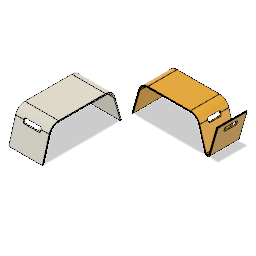
33-Office Desks v1 (Autodesk Fusion 360 design; units mm, degrees)
Autodesk Fusion 360 part; units mm, degrees
sketch "Sketch1" plane through (0, 0, 0) normal (0, 0, 1) x (1, 0, 0)
  line L0 (-100, 0) -> (-84.1445, 55.4944)
  line L1 (-64.914, 70) -> (34.914, 70)
  line L2 (54.1445, 55.4944) -> (68.9639, 3.6264)
  line L3 (73.7715, 0) -> (76.2285, 0)
  line L4 (81.0361, 3.6264) -> (99.8713, 69.5494)
  arc A0 (-64.914, 70) -> (-84.1445, 55.4944) centre (-64.914, 50) ccw
  arc A1 (54.1445, 55.4944) -> (34.914, 70) centre (34.914, 50) ccw
  arc A2 (68.9639, 3.6264) -> (73.7715, 0) centre (73.7715, 5) ccw
  arc A3 (76.2285, 0) -> (81.0361, 3.6264) centre (76.2285, 5) ccw
  line L5 (-102.8846, 0.8242) -> (-87.029, 56.3186)
  arc A4 (-64.914, 73) -> (-87.029, 56.3186) centre (-64.914, 50) ccw
  line L6 (-64.914, 73) -> (34.914, 73)
  arc A5 (57.029, 56.3186) -> (34.914, 73) centre (34.914, 50) ccw
  line L7 (57.029, 56.3186) -> (71.8485, 4.4506)
  arc A6 (71.8485, 4.4506) -> (73.7715, 3) centre (73.7715, 5) ccw
  line L8 (73.7715, 3) -> (76.2285, 3)
  arc A7 (76.2285, 3) -> (78.1515, 4.4506) centre (76.2285, 5) ccw
  line L9 (78.1515, 4.4506) -> (96.9082, 70.0989)
  line L10 (-102.8846, 0.8242) -> (-103.12, 0)
  line L11 (-100, 0) -> (-103.12, 0)
  line L12 (97.8697, 70.8242) -> (98.9097, 70.8242)
  arc A8 (97.8697, 70.8242) -> (96.9082, 70.0989) centre (97.8697, 69.8242) ccw
  arc A9 (99.8713, 69.5494) -> (98.9097, 70.8242) centre (98.9097, 69.8242) ccw
  dimension "d1" = 20
  dimension "d2" = 5
  dimension "d4" = 1
  constraint horizontal L1
  constraint parallel L1 L3
  constraint tangent L0 A0
  constraint tangent L1 A0
  constraint tangent L1 A1
  constraint tangent L2 A1
  constraint equal A0 A1
  constraint tangent L2 A2
  constraint tangent L3 A2
  constraint tangent L3 A3
  constraint tangent L4 A3
  constraint equal A2 A3
  constraint parallel L5 L10
  constraint horizontal L11
  constraint horizontal L12
  constraint parallel L0 L5
  constraint concentric A0 A4
  constraint parallel L1 L6
  constraint concentric A1 A5
  constraint parallel L2 L7
  constraint concentric A2 A6
  constraint parallel L3 L8
  constraint concentric A3 A7
  constraint parallel L4 L9
  constraint tangent A5 L7
  constraint tangent L6 A5
  constraint tangent L5 A4
  constraint tangent A4 L6
  constraint tangent L7 A6
  constraint tangent A6 L8
  constraint tangent L8 A7
  constraint tangent A7 L9
  constraint tangent L9 A8
  constraint tangent L12 A8
  constraint tangent L12 A9
  constraint equal A8 A9
  measures "d1" radius of A0
  measures "d2" radius of A2
  measures "d4" radius of A8
extrude "Extrude1" add sketch "Sketch1" along normal blind 70 makes body 1
sketch "Sketch2" plane through (0, 0, 0) normal (1, 0, 0) x (0, 0, -1)
  line L0 (-22.5, 50) -> (-47.5, 50)
  line L1 (-50, 52.5) -> (-50, 57.5)
  line L2 (-47.5, 60) -> (-22.5, 60)
  line L3 (-20, 57.5) -> (-20, 52.5)
  arc A0 (-47.5, 60) -> (-50, 57.5) centre (-47.5, 57.5) ccw
  arc A1 (-50, 52.5) -> (-47.5, 50) centre (-47.5, 52.5) ccw
  arc A2 (-22.5, 50) -> (-20, 52.5) centre (-22.5, 52.5) ccw
  arc A3 (-20, 57.5) -> (-22.5, 60) centre (-22.5, 57.5) ccw
  dimension "d7" = 2.5
  constraint horizontal L0
  constraint vertical L1
  constraint horizontal L2
  constraint vertical L3
  constraint tangent L1 A0
  constraint tangent L2 A0
  constraint tangent L0 A1
  constraint tangent L1 A1
  constraint equal A0 A1
  constraint tangent L0 A2
  constraint tangent L3 A2
  constraint equal A0 A2
  constraint tangent L2 A3
  constraint tangent L3 A3
  constraint equal A0 A3
  measures "d7" radius of A0
extrude "Extrude2" cut sketch "Sketch2" along normal mid plane 300 bodies 1
fillet "Fillet1" radius 0.5 42 edges at (-95.0745, 28.1593, 0) (-78.7645, 68.362, 0) (-15, 73, 0) (48.7645, 68.362, 0) (64.4387, 30.3846, 0) (72.5671, 3.4033, 0) (75, 3, 0) (77.4329, 3.4033, 0) (87.5299, 37.2747, 0) (97.2675, 70.6225, 0) (98.3897, 70.8242, 0) (99.7081, 70.4264, 0) (90.4537, 36.5879, 0) (79.2395, 1.0083, 0) (75, 0, 0) (70.7605, 1.0083, 0) (61.5542, 29.5604, 0) (46.9579, 65.967, 0) (-15, 70, 0) (-76.9579, 65.967, 0) (-92.0722, 27.7472, 0) (-92.0722, 27.7472, 70) (-76.9579, 65.967, 70) (-15, 70, 70) (46.9579, 65.967, 70) (61.5542, 29.5604, 70) (70.7605, 1.0083, 70) (75, 0, 70) (79.2395, 1.0083, 70) (90.4537, 36.5879, 70) (99.7081, 70.4264, 70) (98.3897, 70.8242, 70) (97.2675, 70.6225, 70) (87.5299, 37.2747, 70) (77.4329, 3.4033, 70) (75, 3, 70) (72.5671, 3.4033, 70) (64.4387, 30.3846, 70) (48.7645, 68.362, 70) (-15, 73, 70) (-78.7645, 68.362, 70) (-95.0745, 28.1593, 70) on bodies 1
sketch "Sketch3" plane through (0, 0, 0) normal (1, 0, 0) x (0, 0, -1)
  line L0 (-220, 0) -> (-204.1445, 55.4944)
  line L1 (-184.914, 70) -> (-74.3884, 70)
  line L2 (-55.158, 55.4944) -> (-39.4041, 0.3558)
  arc A0 (-184.914, 70) -> (-204.1445, 55.4944) centre (-184.914, 50) ccw
  arc A1 (-55.158, 55.4944) -> (-74.3884, 70) centre (-74.3884, 50) ccw
  line L3 (-222.8846, 0.8242) -> (-207.029, 56.3186)
  arc A2 (-184.914, 73) -> (-207.029, 56.3186) centre (-184.914, 50) ccw
  line L4 (-184.914, 73) -> (-74.3884, 73)
  arc A3 (-52.2734, 56.3186) -> (-74.3884, 73) centre (-74.3884, 50) ccw
  line L5 (-52.2734, 56.3186) -> (-36.5195, 1.1799)
  line L6 (-222.8846, 0.8242) -> (-223.12, 0)
  line L7 (-39.4041, 0.3558) -> (-39.3024, 0)
  line L8 (-36.5195, 1.1799) -> (-36.1824, 0)
  line L9 (-223.12, 0) -> (-220, 0)
  line L10 (-39.3024, 0) -> (-36.1824, 0)
  dimension "d12" = 20
  dimension "d13" = 20
  dimension "d14" = -3
  constraint horizontal L1
  constraint tangent L0 A0
  constraint tangent L1 A0
  constraint tangent L1 A1
  constraint tangent L2 A1
  constraint parallel L3 L6
  constraint horizontal L9
  constraint parallel L2 L7
  constraint coincident L7.end L9
  constraint collinear L9 L10
  measures "d12" radius of A0
  measures "d13" radius of A1
extrude "Extrude3" add sketch "Sketch3" against normal blind 80 separate body makes body 2
fillet "Fillet2" radius 0.5 5 edges at (0, 28.1593, 215.0745) (0, 68.362, 198.7645) (0, 73, 129.6512) (0, 68.362, 60.538) (0, 28.1593, 44.2279) on bodies 2
move_body "Move1" bodies 2 to x (1, 0, 0) y (0, 1, 0) z (0, 0, 1) at (-100, 0, 60)
sketch "Sketch4" plane through (0, 0, 0) normal (0, 0, 1) x (1, 0, 0)
  line L0 (-122.5, 50) -> (-157.5, 50)
  line L1 (-160, 52.5) -> (-160, 57.5)
  line L2 (-157.5, 60) -> (-122.5, 60)
  line L3 (-120, 57.5) -> (-120, 52.5)
  arc A0 (-157.5, 60) -> (-160, 57.5) centre (-157.5, 57.5) ccw
  arc A1 (-160, 52.5) -> (-157.5, 50) centre (-157.5, 52.5) ccw
  arc A2 (-122.5, 50) -> (-120, 52.5) centre (-122.5, 52.5) ccw
  arc A3 (-120, 57.5) -> (-122.5, 60) centre (-122.5, 57.5) ccw
  dimension "d19" = 2.5
  constraint horizontal L0
  constraint vertical L1
  constraint horizontal L2
  constraint vertical L3
  constraint tangent L1 A0
  constraint tangent L2 A0
  constraint tangent L0 A1
  constraint tangent L1 A1
  constraint equal A0 A1
  constraint tangent L0 A2
  constraint tangent L3 A2
  constraint equal A0 A2
  constraint tangent L2 A3
  constraint tangent L3 A3
  constraint equal A0 A3
  measures "d19" radius of A0
extrude "Extrude4" cut sketch "Sketch4" along normal blind 380 bodies 2
